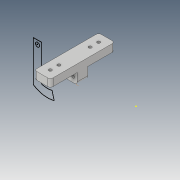
# Autodesk Inventor part: bottomArms
Saved by Autodesk Inventor 2018 (Build 220112000, 112)
## iProperties
Created: 2020-02-27
Part Number: bottomArms
Material: Generic
Document SubType Name: Modeling
Designer: anirudh.bali
Density: 1 g/cm^3
Appearance: Default
Author: anirudh.bali
Autodesk Inventor part; units mm, degrees
ref_plane "YZ Plane" through (0, 0, 0) normal (1, 0, 0) x (0, 1, 0)
ref_plane "XZ Plane" through (0, 0, 0) normal (0, 1, 0) x (-1, 0, 0)
ref_plane "XY Plane" through (0, 0, 0) normal (0, 0, 1) x (1, 0, 0)
sketch "Sketch1" plane through (0, 0, 0) normal (0, 1, 0) x (-1, 0, 0)
  line L0 (69.5198, 0) -> (69.5198, -38.1)
  line L1 (69.5198, -38.1) -> (88.5698, -38.1)
  line L2 (88.5698, -38.1) -> (88.5698, 0)
  line L3 (88.5698, -38.1) -> (69.5198, -38.1)
  line L4 (69.5198, -38.1) -> (69.5198, 38.1)
  line L5 (69.5198, 38.1) -> (88.5698, 38.1)
  line L6 (88.5698, 38.1) -> (88.5698, -38.1)
  line L7 (69.5198, -38.1) -> (88.5698, -38.1)
  line L8 (88.5698, -38.1) -> (88.5698, -19.05)
  line L9 (69.5198, -19.05) -> (69.5198, -38.1)
  circle A0 centre (79.0448, -28.575) radius 1.75
  line L10 (69.5198, 38.1) -> (88.5698, 38.1)
  line L11 (88.5698, 38.1) -> (88.5698, 19.05)
  line L12 (69.5198, 19.05) -> (69.5198, 38.1)
  circle A1 centre (79.0448, 28.575) radius 1.75
  point P0 (0, 0)
  dimension "d0" = 19.05
  dimension "d2" = 19.05
  dimension "d3" = 3.5
  dimension "d4" = 19.05
  dimension "d5" = 3.5
  constraints: 26 end point, 5 parallel, 3 horizontal, 3 perpendicular, 2 centre point, 2 point on line
  measures "d0" distance of L6.end L0.end
  measures "d2" distance of L8.end L8.start
  measures "d3" diameter of A0
  measures "d4" distance of L10.end L11.end
  measures "d5" diameter of A1
ref_plane "Work Plane1" through (-69.5198, 0, 38.1) normal (1, 0, 0) x (0, 0, -1)
sketch "Sketch2" plane through (-69.5198, 0, 38.1) normal (1, 0, 0) x (0, 0, -1)
  line L0 (38.1, 0) -> (31.75, 0)
  line L1 (0, 0) -> (76.2, 0) projected
  line L2 (38.1, 0) -> (44.45, 0)
  line L3 (31.75, 0) -> (26.162, 0)
  line L4 (44.45, 0) -> (50.038, 0)
  line L5 (0, 8.89) -> (76.2, 8.89) projected
  line L6 (31.75, 0) -> (31.75, -8.89)
  line L7 (44.45, -8.89) -> (44.45, 0)
  line L8 (31.75, 0) -> (31.75, -12.7)
  line L9 (31.75, -12.7) -> (44.45, -12.7)
  line L10 (44.45, -12.7) -> (44.45, 0)
  dimension "d26" = 12.7
  constraints: 18 end point, 5 point on line, 2 perpendicular, 1 collinear, 1 vertical
  measures "d26" distance of L0.end L8.end
extrude "Extrusion3" add sketch "Sketch1" along normal blind 8.89
sketch "Sketch3" plane through (0, 8.89, 0) normal (0, 1, 0) x (1, 0, 0)
  circle A0 centre (-79.0448, -28.575) radius 1.75 projected
  circle A1 centre (-79.0448, 28.575) radius 1.75 projected
  circle A2 centre (-79.0448, -18.415) radius 1.75
  circle A3 centre (-79.0448, 18.415) radius 1.75
  point P0 (0, 0)
  dimension "d22" = 3.5
  dimension "d23" = 3.5
  constraints: 2 centre point
  measures "d22" diameter of A2
  measures "d23" diameter of A3
extrude "Extrusion4" cut sketch "Sketch3" against normal blind 18.415 contours A2 | A3
extrude "Extrusion5" add sketch "Sketch2" against normal blind 19.05
sketch "Sketch4" plane through (-69.5198, -12.7, -6.35) normal (0, 0, -1) x (-1, 0, 0)
  line L0 (0, 12.7) -> (0, 0)
  line L1 (19.05, 0) -> (19.05, 12.7) projected
  circle A0 centre (4.7625, 6.35) radius 1.75
  circle A1 centre (14.2875, 6.35) radius 1.75
  point P0 (-69.5198, 12.7)
  dimension "d32" = 3.5
  dimension "d33" = 3.5
  constraints: 2 centre point, 2 end point
  measures "d32" diameter of A0
  measures "d33" diameter of A1
extrude "Extrusion6" cut sketch "Sketch4" against normal blind 19.05
fillet "Fillet1" radius 3.175 6 edges at (-88.5698, 4.445, 38.1) (-69.5198, 4.445, 38.1) (-88.5698, 4.445, -38.1) (-69.5198, 4.445, -38.1) (-88.5698, -12.7, 0) (-69.5198, -12.7, 0)
sketch "Sketch6" plane through (-88.5698, 0, 6.35) normal (0, 0, 1) x (1, 0, 0)
  line L0 (0, 0) -> (0, 8.89) projected
  arc A0 (-32.8405, -38.3954) -> (-8.3696, -42.2273) centre (-16.2814, -12.7) ccw
  line L1 (-10.8348, -33.0268) -> (-8.3696, -42.2273)
  line L2 (-16.2814, -12.7) -> (18.6985, -12.7) construction
  line L3 (-16.2814, -12.7) -> (20.3214, -12.7) construction
  line L4 (-32.8405, 10.0076) -> (-32.8405, -38.3954)
  line L5 (-23.3155, 10.0076) -> (-23.3155, -32.5335)
  arc A1 (-23.3155, -32.5335) -> (-10.8348, -33.0268) centre (-16.2814, -12.7) ccw
  line L6 (-32.8405, 10.0076) -> (-23.3155, 10.0076)
  line L7 (-32.8405, 10.0076) -> (-23.3155, 10.0076)
  line L8 (-23.3155, 10.0076) -> (-23.3155, 0.4826)
  line L9 (-32.8405, 0.4826) -> (-32.8405, 10.0076)
  circle A2 centre (-28.078, 5.2451) radius 2.413
  point P0 (88.5698, 0)
  constraints: 18 end point, 4 horizontal, 4 point on circle, 3 centre point, 2 vertical, 1 coincident, 1 parallel, 1 perpendicular, 1 point on line
body "Solid1"
